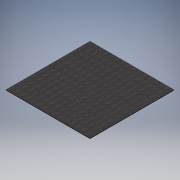
# Autodesk Inventor part: Cement Ground Plane
Saved by Autodesk Inventor 2016 (Build 200138000, 138)
## iProperties
Created: 2015-07-11
Part Number: Cement Ground Plane
Material: Concrete
Document SubType Name: Modeling
Designer: steele
Density: 2.40731 g/cm^3
Appearance: Exposed Aggregate - Coarse
Author: steele
Autodesk Inventor part; units mm, degrees
ref_plane "YZ Plane" through (0, 0, 0) normal (1, 0, 0) x (0, 1, 0)
ref_plane "XZ Plane" through (0, 0, 0) normal (0, 1, 0) x (-1, 0, 0)
ref_plane "XY Plane" through (0, 0, 0) normal (0, 0, 1) x (1, 0, 0)
sketch "Sketch1" plane through (0, 0, 0) normal (0, 1, 0) x (-1, 0, 0)
  line L0 (-1371.6, 1371.6) -> (-1371.6, -1371.6)
  line L1 (-1371.6, -1371.6) -> (1371.6, -1371.6)
  line L2 (1371.6, -1371.6) -> (1371.6, 1371.6)
  line L3 (1371.6, 1371.6) -> (-1371.6, 1371.6)
  line L4 (-1371.6, 1371.6) -> (1371.6, -1371.6) construction
  line L5 (-1371.6, -1371.6) -> (1371.6, 1371.6) construction
  point P0 (0, 0)
  dimension "d0" = 2743.2
  constraints: 12 end point, 2 midpoint, 2 parallel, 2 perpendicular, 1 vertical
  measures "d0" distance of L0.end L1.end
extrude "Extrusion1" add sketch "Sketch1" against normal blind 25.4
body "Solid1"
